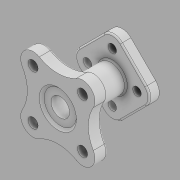
# Autodesk Inventor part: Lab6A01209499P2
Saved by Autodesk Inventor 2020 (Build 240168000, 168)
## iProperties
Created: 2019-10-03
Part Number: Lab6A01209499P2
Material: Genérico
Document SubType Name: Modeling
Designer: gerar
Density: 1 g/cm^3
Appearance: Valor por defecto
Author: gerar
Autodesk Inventor part; units mm, degrees
ref_plane "YZ Plane" through (0, 0, 0) normal (1, 0, 0) x (0, 1, 0)
ref_plane "XZ Plane" through (0, 0, 0) normal (0, 1, 0) x (-1, 0, 0)
ref_plane "XY Plane" through (0, 0, 0) normal (0, 0, 1) x (1, 0, 0)
sketch "Boceto3" plane through (0, 0, 0) normal (0, 0, 1) x (1, 0, 0)
  line L0 (-53.34, 0) -> (53.34, 0) construction
  line L1 (0, -53.34) -> (0, 53.34) construction
  line L2 (0, -25.4) -> (25.4, 0) construction
  line L3 (25.4, 0) -> (0, 25.4) construction
  line L4 (0, 25.4) -> (-25.4, 0) construction
  line L5 (-25.4, 0) -> (0, -25.4) construction
  line L6 (0, -25.4) -> (0, 25.4) construction
  line L7 (25.4, 0) -> (-25.4, 0) construction
  arc A0 (-34.3803, 8.9803) -> (-34.3803, -8.9803) centre (-25.4, 0) ccw
  arc A1 (8.9803, 34.3803) -> (-8.9803, 34.3803) centre (0, 25.4) ccw
  arc A2 (34.3803, -8.9803) -> (34.3803, 8.9803) centre (25.4, 0) ccw
  arc A3 (-8.9803, -34.3803) -> (8.9803, -34.3803) centre (0, -25.4) ccw
  circle A4 centre (-25.4, 0) radius 4.3688
  circle A5 centre (0, 25.4) radius 4.3688
  circle A6 centre (25.4, 0) radius 4.3688
  circle A7 centre (0, -25.4) radius 4.3688
  line L8 (-34.3803, 8.9803) -> (-8.9803, 34.3803)
  line L9 (8.9803, 34.3803) -> (34.3803, 8.9803)
  line L10 (34.3803, -8.9803) -> (8.9803, -34.3803)
  line L11 (-8.9803, -34.3803) -> (-34.3803, -8.9803)
  point P0 (0, 0)
  dimension "d30" = 25.4
  dimension "d31" = 50.8
  dimension "d32" = 50.8
  dimension "d33" = 25.4
  dimension "d34" = 12.7
  dimension "d35" = 12.7
  dimension "d36" = 12.7
  dimension "d37" = 12.7
  dimension "d38" = 8.7376
  dimension "d39" = 8.7376
  dimension "d40" = 8.7376
  dimension "d41" = 8.7376
  constraints: 20 end point, 8 centre point, 8 coincident, 8 point on circle, 5 tangent, 4 perpendicular, 2 parallel
  measures "d30" distance of point (0, 0) L3.end
  measures "d31" distance of L2.start L3.end
  measures "d32" distance of L2.end L4.end
  measures "d33" distance from line of L1 L4.end
  measures "d34" radius of A3
  measures "d35" radius of A1
  measures "d36" radius of A2
  measures "d37" radius of A0
  measures "d38" diameter of A4
  measures "d39" diameter of A7
  measures "d40" diameter of A6
  measures "d41" diameter of A5
extrude "Base" add sketch "Boceto3" along normal blind 10.16
sketch "Boceto4" plane through (0, 0, 10.16) normal (0, 0, 1) x (1, 0, 0)
  circle A0 centre (0, 0) radius 13.97
  dimension "d44" = 27.94
  constraints: 1 centre point, 1 coincident
  measures "d44" diameter of A0
extrude "Cilindro" add sketch "Boceto4" along normal blind 55.88
sketch "Boceto5" plane through (0, 0, 66.04) normal (0, 0, 1) x (1, 0, 0)
  line L0 (-25.4, -25.4) -> (25.4, -25.4) construction
  line L1 (25.4, -25.4) -> (25.4, 25.4) construction
  line L2 (25.4, 25.4) -> (-25.4, 25.4) construction
  line L3 (-25.4, 25.4) -> (-25.4, -25.4) construction
  line L4 (-25.4, -25.4) -> (25.4, 25.4) construction
  line L5 (25.4, -25.4) -> (-25.4, 25.4) construction
  arc A0 (-19.05, 36.3985) -> (-36.3985, 19.05) centre (-25.4, 25.4) ccw
  arc A1 (-36.3985, -19.05) -> (-19.05, -36.3985) centre (-25.4, -25.4) ccw
  arc A2 (19.05, -36.3985) -> (36.3985, -19.05) centre (25.4, -25.4) ccw
  arc A3 (36.3985, 19.05) -> (19.05, 36.3985) centre (25.4, 25.4) ccw
  circle A4 centre (-25.4, 25.4) radius 5.1562
  circle A5 centre (-25.4, -25.4) radius 5.1562
  circle A6 centre (25.4, -25.4) radius 5.1562
  circle A7 centre (25.4, 25.4) radius 5.1562
  arc A8 (-36.3985, -19.05) -> (-36.3985, 19.05) centre (-69.3941, 0) ccw
  arc A9 (-19.05, 36.3985) -> (19.05, 36.3985) centre (0, 69.3941) ccw
  arc A10 (36.3985, 19.05) -> (36.3985, -19.05) centre (69.3941, 0) ccw
  arc A11 (19.05, -36.3985) -> (-19.05, -36.3985) centre (0, -69.3941) ccw
  point P0 (0, 0)
  dimension "d47" = 50.8
  dimension "d48" = 50.8
  dimension "d49" = 25.4
  dimension "d50" = 25.4
  dimension "d51" = 25.4
  dimension "d52" = 25.4
  dimension "d53" = 10.3124
  dimension "d54" = 10.3124
  dimension "d55" = 10.3124
  dimension "d56" = 10.3124
  dimension "d57" = 25.4
  dimension "d58" = 76.2
  dimension "d59" = 76.2
  dimension "d60" = 76.2
  dimension "d61" = 76.2
  constraints: 16 point on circle, 12 centre point, 12 end point, 8 coincident, 8 tangent, 2 midpoint, 2 parallel, 1 horizontal, 1 perpendicular
  measures "d47" distance of L2.end L1.end
  measures "d48" distance of L1.end L0.end
  measures "d49" diameter of A0
  measures "d50" diameter of A1
  measures "d51" diameter of A2
  measures "d52" diameter of A3
  measures "d53" diameter of A4
  measures "d54" diameter of A5
  measures "d55" diameter of A6
  measures "d56" diameter of A7
  measures "d57" horizontal distance of point (0, 0) L2.end
  measures "d58" diameter of A8
  measures "d59" diameter of A9
  measures "d60" diameter of A10
  measures "d61" diameter of A11
extrude "Extrusión5" add sketch "Boceto5" against normal blind 12.7
sketch "Boceto6" plane through (0, 0, 66.04) normal (0, 0, 1) x (1, 0, 0)
  point P0 (0, 0)
  point P1 (0, 0)
  constraints: 1 coincident
hole "Agujero1" at (0, 0, 66.04) direction (0, 0, -1) diameter 19.05 depth 38.1 counterbore diameter 38.1 counterbore depth 2.54
draft "Cara para el ángulo de desmoldeo1" angle 45 pull direction (0, 0, 1) faces at (1.5329, -18.9882, 65.1933) fixed edges at (0, 19.05, 66.04)
fillet "Empalme1" radius 1.524 17 edges at (0, 38.1, 10.16) (-21.6803, 21.6803, 10.16) (-38.1, 0, 10.16) (-21.6803, -21.6803, 10.16) (0, -38.1, 10.16) (21.6803, -21.6803, 10.16) (38.1, 0, 10.16) (21.6803, 21.6803, 10.16) (-13.97, 0, 10.16) (34.3803, 34.3803, 53.34) (31.2941, 0, 53.34) (34.3803, -34.3803, 53.34) (0, -31.2941, 53.34) (-34.3803, -34.3803, 53.34) (-31.2941, 0, 53.34) (-34.3803, 34.3803, 53.34) (0, 31.2941, 53.34)
